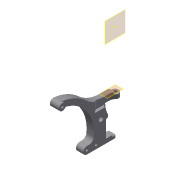
# Autodesk Inventor part: thumb_base
Saved by Autodesk Inventor 2014 (Build 180170000, 170)
## iProperties
Created: 2015-05-30
Part Number: thumb_base
Material: Generic
Document SubType Name: Modeling
Designer: Martin
Density: 1 g/cm^3
Appearance: Default
Author: Martin
Autodesk Inventor part; units mm, degrees
ref_plane "YZ Plane" through (0, 0, 0) normal (1, 0, 0) x (0, 1, 0)
ref_plane "XZ Plane" through (0, 0, 0) normal (0, 1, 0) x (-1, 0, 0)
ref_plane "plane_main" through (10, -20, 0) normal (1, 0, 0) x (0, 1, 0)
sketch "Sketch1" plane through (10, -20, 0) normal (1, 0, 0) x (0, 1, 0)
  line L0 (0, -108) -> (0, 18)
  line L1 (20, -86.5) -> (15.45, -86.5) projected
  line L2 (-1.875, -97.5779) -> (1.875, -97.5779) projected
  line L3 (-2.5, -63.4852) -> (2.5, -63.4852) projected
  line L4 (4, -96.0779) -> (-9.3, -96.0779)
  line L5 (-9.3, -96.0779) -> (-9.3, -62.9852)
  line L6 (-9.3, -62.9852) -> (4, -62.9852)
  line L7 (4, -62.9852) -> (4, -58.4852)
  line L8 (4, -58.4852) -> (-13.4946, -58.4852)
  line L9 (-13.4946, -58.4852) -> (-19.3, -92.5779)
  line L10 (-19.3, -92.5779) -> (-34.3, -92.5779)
  line L11 (-34.3, -92.5779) -> (-34.3, -100.5779) construction
  line L12 (-34.3, -100.5779) -> (4, -100.5779)
  line L13 (4, -96.0779) -> (4, -100.5779)
  line L14 (-7.3, -76.7852) -> (-7.3, -63.4852) projected
  arc A0 (-34.3, -92.5779) -> (-34.3, -100.5779) centre (-34.3, -96.5779) ccw
  circle A1 centre (-34.3, -96.5779) radius 1.25
  circle A2 centre (-24.3, -96.5779) radius 1.25
  line L15 (-34.3, -96.5779) -> (-24.3, -96.5779) construction
  point P0 (20, 0)
  dimension "d0" = 0.5
  dimension "d1" = 1.5
  dimension "d2" = 4.5
  dimension "d3" = 4.5
  dimension "d4" = 8
  dimension "d7" = 33.0927
  dimension "d8" = 2.5
  dimension "d9" = 10
  dimension "d10" = 15
  dimension "d11" = 10
  dimension "d12" = 2
  dimension "d21" = 4
  dimension "d22" = 4
  constraints: 24 end point, 7 perpendicular, 4 parallel, 3 centre point, 2 point on circle, 2 tangent, 1 coincident, 1 equal radius, 1 vertical, 2 other
  measures "d0" distance between parallel lines of L6 L3
  measures "d1" distance between parallel lines of L4 L2
  measures "d2" distance of L6.end L7.end
  measures "d3" distance between parallel lines of L4 L12
  measures "d4" distance between parallel lines of L12 L10
  measures "d7" distance of L4.end L5.end
  measures "d8" diameter of A1
  measures "d9" distance of L15.start L15.end
  measures "d10" horizontal distance of L9.end A0.centre
  measures "d11" horizontal distance of L4.end L9.end
  measures "d12" distance between parallel lines of L14 L5
  measures "d21" distance between parallel lines of L0 L7
  measures "d22" distance between parallel lines of L0 L13
extrude "ext_main" add sketch "Sketch1" along normal mid plane 8 contours L12 A0 L10 L9 L8 L0 L6 L5 L4 | L0 L4 L13 L12 | L0 L8 L7 L6
fillet "Fillet1" radius 2 3 edges at (10, -39.3, -92.5779) (10, -33.4946, -58.4852) (10, -29.3, -96.0779)
sketch "Sketch3" plane through (6, -16, -58.4852) normal (0, 0, 1) x (1, 0, 0)
  circle A0 centre (4, -3.2197) radius 1.5
  point P0 (-6, 16)
  dimension "d17" = 3
  constraints: 1 centre point, 1 coincident, 1 other
  measures "d17" diameter of A0
extrude "ext_cut_topbore" cut sketch "Sketch3" against normal up to surface (4.5 mm away)
fillet "Fillet2" radius 4 4 edges at (14, -16, -60.7352) (6, -16, -60.7352) (14, -16, -98.3279) (6, -16, -98.3279)
ref_plane "Work Plane2" through (6, -31.8064, -58.4852) normal (0, 0, 1) x (1, 0, 0)
sketch "Sketch5" plane through (6, -31.8064, -58.4852) normal (0, 0, 1) x (1, 0, 0)
  line L0 (8, 11.8064) -> (8, 0) projected
  circle A0 centre (14, 4.111) radius 9
  circle A1 centre (4, 12.5867) radius 1.5 projected
  arc A2 (8, 11.8064) -> (0, 11.8064) centre (4, 11.8064) ccw projected
  arc A3 (7.3747, 10.2024) -> (8, 11.8064) centre (5.6301, 11.8064) ccw
  line L1 (8, 11.8064) -> (8, 10.8192)
  line L2 (5, 4.111) -> (5, -4.889)
  line L3 (5, -4.889) -> (14, -4.889)
  point P0 (-6, 31.8064)
  point P1 (4, 12.611)
  dimension "d27" = 18
  dimension "d28" = 8.5
  dimension "d29" = 10
  constraints: 6 end point, 6 point on circle, 4 tangent, 2 centre point, 1 parallel, 1 perpendicular, 1 point on line, 1 other
  measures "d27" diameter of A0
  measures "d28" vertical distance of point (4, 12.611) A0.centre
  measures "d29" horizontal distance of point (4, 12.611) A0.centre
extrude "ext_cut_motor_cutway" cut sketch "Sketch5" along normal mid plane 15 contours L0 A0 A3 | A0 | A0 L3 L2
fillet "Fillet4" [suppressed]
sketch "Sketch6" plane through (10, -20, 0) normal (1, 0, 0) x (0, 1, 0)
  line L0 (0, -96.0779) -> (0, -96.0779) projected
  line L1 (-7.3, -96.0779) -> (0, -96.0779) projected
  line L2 (0, -96.0779) -> (-7.3, -96.0779) projected
  line L3 (0, -100.5779) -> (0, -100.5779) projected
  line L4 (-34.3, -100.5779) -> (0, -100.5779) projected
  line L5 (0, -100.5779) -> (-34.3, -100.5779) projected
  line L6 (0.7803, -108) -> (0.7803, 18) construction
  line L7 (0.7803, -96.0779) -> (0.7803, -100.5779)
  line L8 (1.5303, -100.5779) -> (1.5303, -98.2779)
  line L9 (1.5303, -98.2779) -> (2.7803, -98.2779)
  line L10 (2.7803, -98.2779) -> (2.7803, -96.0779)
  line L11 (2.7803, -96.0779) -> (0.7803, -96.0779)
  line L12 (0, -96.0779) -> (-7.3, -96.0779) projected
  line L13 (0.7803, -100.5779) -> (1.5303, -100.5779)
  line L14 (-34.3, -100.5779) -> (0, -100.5779) projected
  point P0 (20, 0)
  dimension "d37" = 0.75
  dimension "d38" = 2
  dimension "d39" = 2.2
  constraints: 14 end point, 4 parallel, 4 point on line, 1 perpendicular, 1 vertical, 2 other
  measures "d37" distance between parallel lines of L6 L8
  measures "d38" distance between parallel lines of L6 L10
  measures "d39" distance between parallel lines of L11 L9
revolve "revolution_servohubfit" cut sketch "Sketch6" angle 360 about axis through (10, -19.2197, -108) along (0, 0, 1)
sketch "Sketch7" plane through (10, -20, 0) normal (1, 0, 0) x (0, 1, 0)
  line L0 (0, -100.5779) -> (0, -96.0779) projected
  line L1 (0, -100.5779) -> (-34.3, -100.5779) projected
  arc A0 (-34.3, -92.5779) -> (-34.3, -100.5779) centre (-34.3, -96.5779) ccw projected
  line L2 (-34.3, -92.5779) -> (-20.9882, -92.5779) projected
  arc A1 (-20.9882, -92.5779) -> (-19.0166, -90.9136) centre (-20.9882, -90.5779) ccw projected
  line L3 (-19.0166, -90.9136) -> (-13.778, -60.1495) projected
  arc A2 (-11.8064, -58.4852) -> (-13.778, -60.1495) centre (-11.8064, -60.4852) ccw projected
  line L4 (-11.8064, -58.4852) -> (0, -58.4852) projected
  line L5 (0, -62.9852) -> (0, -58.4852) projected
  line L6 (0, -62.9852) -> (-9.3, -62.9852) projected
  line L7 (-9.3, -62.9852) -> (-9.3, -94.0779) projected
  arc A3 (-9.3, -94.0779) -> (-7.3, -96.0779) centre (-7.3, -94.0779) ccw projected
  line L8 (-7.3, -96.0779) -> (0, -96.0779) projected
  circle A4 centre (-34.3, -96.5779) radius 1.25 projected
  circle A5 centre (-24.3, -96.5779) radius 1.25 projected
  line L9 (-34.3, -96.5779) -> (-24.3, -96.5779)
  line L10 (-24.3, -96.5779) -> (-24.3, -86.5779)
  line L11 (-24.3, -86.5779) -> (-62.8673, -40.6152) construction
  line L12 (-24.3, -86.5779) -> (-34.3, -96.5779) construction
  circle A6 centre (-62.8673, -40.6152) radius 1.25
  arc A7 (-24.3, -86.5779) -> (-62.8673, -40.6152) centre (-67.714, -83.8444) ccw construction
  line L13 (-34.3911, -55.8831) -> (-43.5836, -63.5965) construction
  circle A8 centre (-62.8673, -40.6152) radius 3.75
  line L14 (-19.0166, -90.9136) -> (-13.778, -60.1495) projected
  arc A9 (-24.3, -86.5779) -> (-59.1621, -41.1933) centre (-67.714, -83.8444) ccw
  arc A10 (-27.6511, -92.5779) -> (-60.4568, -43.4879) centre (-67.714, -83.8444) ccw
  line L15 (-19.2968, -92.5591) -> (-19.2968, -100.5779)
  line L16 (-24.3, -92.5779) -> (-24.3, -95.3279)
  line L17 (-19.2968, -95.3279) -> (-24.3, -95.3279)
  arc A11 (-21.1977, -75.5502) -> (-16.3973, -75.5315) centre (-18.7991, -75.1225) ccw
  line L18 (-14.7717, -65.9852) -> (-19.0166, -90.9136) projected
  arc A12 (-62.0154, -36.9632) -> (-62.0154, -36.9632) centre (-74.2254, -89.308) ccw
  arc A13 (-21.2777, -92.5754) -> (-62.4494, -36.8886) centre (-67.714, -83.8444) ccw
  point P0 (20, 0)
  point P1 (-15.2647, -70.072)
  dimension "d41" = 60
  dimension "d43" = 10
  dimension "d44" = 140
  dimension "d45" = 2.5
  dimension "d46" = 12
  dimension "d53" = 2.5
  constraints: 19 point on circle, 16 end point, 8 centre point, 7 point on line, 4 perpendicular, 3 concentric, 2 coincident, 2 midpoint, 2 tangent, 1 horizontal, 1 line through centre, 1 parallel, 1 vertical alignment, 5 other
  measures "d41" distance of L10.end L11.end
  measures "d43" distance of L9.end L10.end
  measures "d44" angle of L10 L11
  measures "d45" diameter of A6
  measures "d46" distance of L13.start L13.end
  measures "d53" radial gap between concentric circles of A6 A8
extrude "ext_thumbbevel" add sketch "Sketch7" along normal mid plane 8 contours A13 A12 | A12 A8 A13 | A12 A1 L2 L10 A9 A8 | A8 | A11 L3 A1 A12 A13 | A10 A8 A9 L10 L2
fillet "Fillet7" radius 5 2 edges at (10, -80.4568, -43.4879) (10, -47.6511, -92.5779)
sketch "Sketch11" plane through (6, -20, 0) normal (-1, 0, 0) x (0, 0, 1)
  circle A0 centre (-40.6152, -62.8673) radius 1.25 projected
  arc A1 (-44.1033, -61.4905) -> (-36.8886, -62.4494) centre (-40.6152, -62.8673) ccw projected
  line L0 (-96.0779, -7.3) -> (-96.0779, 0) projected
  circle A2 centre (-40.6152, -62.8673) radius 2
  line L1 (-42.6152, -62.8673) -> (-38.6152, -62.8673) construction
  line L2 (-120.6935, 20) -> (20.1156, 20) projected
  line L3 (-42.0435, -61.4673) -> (-39.1869, -61.4673)
  line L4 (-42.0435, -64.2673) -> (-39.1869, -64.2673)
  point P0 (0, 20)
  dimension "d68" = 4
  dimension "d69" = 2.8
  constraints: 6 end point, 6 point on circle, 3 parallel, 2 symmetric about line, 1 centre point, 1 coincident, 1 midpoint, 1 perpendicular
  measures "d68" diameter of A2
  measures "d69" distance between parallel lines of L4 L3
extrude "ext_cut_potshaft" cut sketch "Sketch11" against normal blind 5.75 contours A0 | A2 L4 L3
sketch "Sketch12" plane through (14, -20, 0) normal (1, 0, 0) x (0, 0, -1)
  circle A0 centre (40.6152, -62.8673) radius 1.25 projected
  arc A1 (36.8886, -62.4494) -> (44.1033, -61.4905) centre (40.6152, -62.8673) ccw projected
  circle A2 centre (40.6152, -62.8673) radius 3.75
  point P0 (0, 20)
  constraints: 1 centre point, 1 coincident, 1 concentric
extrude "ext_screwextension" add sketch "Sketch12" along normal blind 2
sketch "Sketch15" plane through (6, -20, 0) normal (-1, 0, 0) x (0, 0, 1)
  arc A0 (-36.8886, -62.4494) -> (-75.5502, -21.1977) centre (-83.8444, -67.714) ccw projected
  arc A1 (-75.5315, -16.3973) -> (-75.5502, -21.1977) centre (-75.1225, -18.7991) ccw projected
  line L0 (-75.5315, -16.3973) -> (-60.1495, -13.778) projected
  arc A2 (-60.1495, -13.778) -> (-58.4852, -11.8064) centre (-60.4852, -11.8064) ccw projected
  line L1 (-58.4852, -11.8064) -> (-58.4852, 0) projected
  arc A3 (-58.4852, -11.8064) -> (-49.1566, -35.631) centre (-23.3977, -11.8064) ccw
  circle A4 centre (-75.1225, -18.7991) radius 2.4364
  line L2 (-75.5315, -16.3973) -> (-60.1495, -13.778)
  arc A5 (-60.1495, -13.778) -> (-58.4852, -11.8064) centre (-60.4852, -11.8064) ccw
  arc A6 (-49.1566, -35.631) -> (-75.5502, -21.1977) centre (-83.8444, -67.714) ccw
  point P0 (0, 20)
  constraints: 9 tangent, 7 point on circle, 4 centre point, 2 end point, 1 coincident, 1 collinear, 1 concentric
extrude "ext_bevelfill" add sketch "Sketch15" against normal blind 8 contours A0 A4 L0 A2 A3
sketch "Sketch16" plane through (6, -31.8064, -58.4852) normal (0, 0, 1) x (1, 0, 0)
  line L0 (8, -2.9653) -> (5, -2.9653) projected
  line L1 (8, 2.5064) -> (8, -2.9653) projected
  line L2 (5, 2.5064) -> (8, 2.5064) projected
  line L3 (5, -2.9653) -> (5, 2.5064) projected
  line L4 (8, 0) -> (8, -23.8246) projected
  line L5 (5, -2.9653) -> (5, -7.9972)
  arc A0 (5, -7.9972) -> (8, -13.6434) centre (11.8132, -7.9972) ccw
  line L6 (8, -13.6434) -> (8, -2.9653)
  line L7 (8, -2.9653) -> (5, -2.9653)
  point P0 (-6, 31.8064)
  constraints: 6 end point, 2 point on circle, 1 centre point, 1 collinear, 1 parallel, 1 perpendicular, 1 point on line, 1 tangent
extrude "ext_cut_cutway_WORKAROUND" cut sketch "Sketch16" against normal blind 7.5 and the other way blind 4
sketch "Sketch18" plane through (0, 0, 0) normal (1, 0, 0) x (0, 1, 0)
  line L0 (-29.3, -62.9852) -> (-29.3, -65.9852) projected
  line L1 (-29.3, -94.0779) -> (-29.3, -65.9852) projected
  line L2 (-29.3, -62.9852) -> (-29.3, -94.0779) projected
  line L3 (-20, -96.0779) -> (-27.3, -96.0779) projected
  line L4 (-29.3, -96.0779) -> (-29.3, -62.9852)
  line L5 (-29.3, -62.9852) -> (-31.55, -62.9852)
  line L6 (-31.55, -62.9852) -> (-31.55, -76.7788)
  line L7 (-31.55, -76.7788) -> (-33.8, -78.0779)
  line L8 (-33.8, -78.0779) -> (-33.8, -96.0779)
  line L9 (-33.8, -96.0779) -> (-29.3, -96.0779)
  line L10 (-27.3, -96.0779) -> (-29.3, -94.0779)
  line L11 (-29.3, -96.0779) -> (-27.3, -96.0779)
  point P0 (0, 0)
  dimension "d88" = 120
  dimension "d89" = 18
  dimension "d90" = 2.25
  dimension "d91" = 4.5
  constraints: 16 end point, 3 collinear, 2 parallel, 2 perpendicular
  measures "d88" angle of L6 L7
  measures "d89" distance of L7.end L8.end
  measures "d90" distance between parallel lines of L1 L6
  measures "d91" distance of L8.end L4.start
extrude "ext_cut_xtrainnerspace" cut sketch "Sketch18" along normal through all
sketch "sk_servohub_clamp" plane through (14, -54.3, -100.5779) normal (0, 0, -1) x (-1, 0, 0)
  circle A0 centre (4, 35.0803) radius 0.75 projected
  arc A1 (8, 34.3) -> (0, 34.3) centre (4, 34.3) ccw projected
  line L0 (8, 34.3) -> (8, 0) projected
  line L1 (4, 35.0803) -> (4, 43.0803) construction
  line L2 (0, 34.3) -> (0, 39.0803)
  line L3 (0, 39.0803) -> (8, 39.0803) construction
  line L4 (8, 39.0803) -> (8, 34.3)
  arc A2 (8, 39.0803) -> (0, 39.0803) centre (4, 39.0803) ccw
  line L5 (3.4, 43.035) -> (3.4, 30.0803)
  line L6 (3.4, 30.0803) -> (4.6, 30.0803) construction
  line L7 (4.6, 30.0803) -> (4.6, 43.035)
  arc A3 (3.4, 30.0803) -> (4.6, 30.0803) centre (4, 30.0803) ccw
  line L8 (4, 35.0803) -> (4, 30.0803) construction
  arc A4 (3.4, 38.2547) -> (0, 34.3) centre (4, 34.3) ccw
  arc A5 (8, 34.3) -> (4.6, 38.2547) centre (4, 34.3) ccw
  line L9 (3.4, 38.2547) -> (3.4, 43.035)
  line L10 (4.6, 43.035) -> (4.6, 38.2547)
  point P0 (14, 54.3)
  dimension "d94" = 1.2
  dimension "d95" = 5
  dimension "d96" = 4
  constraints: 20 end point, 14 point on circle, 5 tangent, 4 centre point, 4 collinear, 4 parallel, 2 concentric, 2 perpendicular, 1 point on line
  measures "d94" distance between parallel lines of L7 L5
  measures "d95" distance from line of L1.start L6
  measures "d96" distance from line of L1.start L3
extrude "ext_servoclamp" [suppressed]
extrude "ext_cut_servoclamt_slot" [suppressed]
sketch "Sketch21" plane through (14, -20, 0) normal (1, 0, 0) x (0, 0, -1)
  point P0 (0, 20)
extrude "ext_cut_servoclampscrew" [suppressed]
sketch "Sketch24" plane through (14, -54.3, -100.5779) normal (0, 0, -1) x (-1, 0, 0)
  circle A0 centre (4, 35.0803) radius 0.75 projected
  arc A1 (8, 34.3) -> (0, 34.3) centre (4, 34.3) ccw projected
  line L0 (0, 0) -> (0, 34.3) projected
  line L1 (8, 0) -> (0, 0) projected
  line L2 (8, 34.3) -> (8, 0) projected
  circle A2 centre (4, 35.0803) radius 3.5
  line L3 (0, 31.5803) -> (8, 31.5803)
  arc A3 (1.1367, 37.0931) -> (0, 34.3) centre (4, 34.3) ccw
  arc A4 (8, 34.3) -> (6.8633, 37.0931) centre (4, 34.3) ccw
  line L4 (0, 31.5803) -> (0, 34.3)
  line L5 (8, 31.5803) -> (8, 34.3)
  line L6 (4, 35.0803) -> (4, 20.1803) construction
  circle A5 centre (4, 28.1303) radius 0.5
  circle A6 centre (4, 22.2303) radius 0.5
  circle A7 centre (4, 35.0803) radius 1.95 construction
  point P0 (14, 54.3)
  point P1 (4, 27.6303)
  point P2 (4, 37.0303)
  dimension "d117" = 3.9
  dimension "d114" = 7
  dimension "d115" = 1
  dimension "d116" = 5.9
  dimension "d118" = 9.4
  constraints: 9 point on circle, 8 end point, 7 tangent, 5 point on line, 4 centre point, 3 coincident, 2 collinear, 2 concentric, 2 vertical alignment, 1 midpoint, 1 parallel, 1 perpendicular, 5 other
  measures "d114" diameter of A2
  measures "d115" diameter of A6
  measures "d116" distance of A6.centre point (4, 28.13)
  measures "d118" distance of point (4, 37.03) point (4, 27.63)
extrude "ext_cut_servohubfit" cut sketch "Sketch24" against normal up to surface (4.5 mm away) contours L2 L3 A2 A1 | A2 A1 | A1 A2 | A2 L3 L0 A1 | A5 | A6
fillet "Fillet8" radius 1 2 edges at (14, -22.7197, -98.3279) (6, -22.7197, -98.3279)
sketch "Sketch25" plane through (10, -20, -62.9852) normal (0, 0, -1) x (-1, 0, 0)
  circle A0 centre (0, 0.7803) radius 1.5 projected
  arc A1 (-4, 0) -> (-3.3747, -1.604) centre (-1.6301, 0) ccw projected
  arc A2 (-1, -7.6954) -> (-3.3747, -1.604) centre (-10, -7.6954) ccw projected
  line L0 (-1, -11.55) -> (-1, -7.6954) projected
  line L1 (4, -11.55) -> (-1, -11.55) projected
  line L2 (4, 0) -> (4, -11.55) projected
  arc A3 (4, 0) -> (-4, 0) centre (0, 0) ccw projected
  point P0 (10, 20)
extrude "Extrusion24" add sketch "Sketch25" along normal blind 2
sketch "Sketch26" plane through (10, -20, -58.4852) normal (0, 0, 1) x (1, 0, 0)
  arc A0 (3.3747, -1.604) -> (4, 0) centre (1.6301, 0) ccw projected
  arc A1 (4, 0) -> (-4, 0) centre (0, 0) ccw projected
  line L0 (-4, -11.8064) -> (-4, 0) projected
  arc A2 (3.3747, -1.604) -> (1, -7.6954) centre (10, -7.6954) ccw projected
  circle A3 centre (0, 0.7803) radius 1.5 projected
  circle A4 centre (0, 0.7803) radius 3.25
  line L1 (0, -2.4697) -> (-4, -2.4697)
  line L2 (0, -2.4697) -> (2.6725, -2.4697)
  point P0 (-10, 20)
  dimension "d124" = 6.5
  constraints: 4 end point, 1 coincident, 1 collinear, 1 horizontal, 1 perpendicular, 1 point on circle, 1 point on line, 1 vertical alignment, 2 other
extrude "Extrusion25" cut sketch "Sketch26" against normal blind 2.2 contours A2 L2 A4 A1 A0 | A4 A1 | L1 L0 A1 A4 picked at (-1.0722, 3.2045)
fillet "Fillet9" radius 1 2 edges at (12.6725, -22.4697, -59.5852) (6, -22.4697, -59.5852)
sketch "Sketch27" plane through (10, -20, 0) normal (1, 0, 0) x (0, 1, 0)
  line L0 (-2.7197, -96.0779) -> (-6.7197, -96.0779)
  line L1 (-6.7197, -96.0779) -> (-6.7197, -97.7779)
  line L2 (-6.7197, -97.7779) -> (-2.7197, -97.7779)
  line L3 (-2.7197, -97.7779) -> (-2.7197, -96.0779)
  point P0 (20, 0)
  dimension "d128" = 1.7
  dimension "d129" = 4
  constraints: 8 end point, 2 parallel, 1 horizontal, 1 perpendicular
  measures "d128" distance of L2.end L0.start
  measures "d129" distance of L0.start L0.end
extrude "Extrusion26" cut sketch "Sketch27" along normal through all both and the other way through all
sketch "Sketch28" plane through (6, -31.55, -76.7788) normal (0, 1, 0) x (1, 0, 0)
  line L0 (5, -10.7936) -> (5, -11.7936) projected
  line L1 (8, -10.7936) -> (5, -10.7936) projected
  line L2 (8, 0) -> (8, -10.7936) projected
  arc A0 (8, -2.7936) -> (5, -10.7936) centre (17.1667, -10.7936) ccw
  line L3 (5, -10.7936) -> (8, -10.7936)
  line L4 (8, -2.7936) -> (8, -10.7936)
  point P0 (-6, -76.7788)
  dimension "d132" = 8
  constraints: 4 end point, 2 collinear, 2 point on circle, 1 centre point, 1 point on line, 1 tangent
  measures "d132" distance from line of L1 L4.start
revolve "Revolution2" cut sketch "Sketch28" angle 360 about axis through (14, -31.55, -76.7788) along (0, 0, 1)
equation "\"d8\" = screw_m2_bore_loose"
equation "\"d21\" = 0.5 * model_main_thickness"
equation "\"d22\" = 0.5 * model_main_thickness"
equation "\"d5\" = model_main_thickness"
equation "\"d17\" = screw_m3_bore_selfthreading"
equation "\"d20\" = 0.5 * model_main_thickness"
equation "\"d36\" = 0.5 * model_main_thickness"
equation "\"d37\" = 0.5 * model_servoscrew_diam"
equation "\"d38\" = 0.5 * model_servohub_diam"
equation "\"d45\" = screw_m2_bore_loose"
equation "\"d54\" = model_main_thickness"
equation "\"d76\" = model_main_thickness"
equation "\"d94\" = 3 * print_support_z_clearance"
equation "\"model_main_thickness\" = 8"
equation "\"model_servoscrew_diam\" = 1.5"
equation "\"model_servohub_diam\" = 4"
equation "\"screw_m2_bore_loose\" = 2.5"
equation "\"screw_m3_bore_selfthreading\" = 3"
equation "\"print_support_z_clearance\" = 0.4"
body "Solid1"
